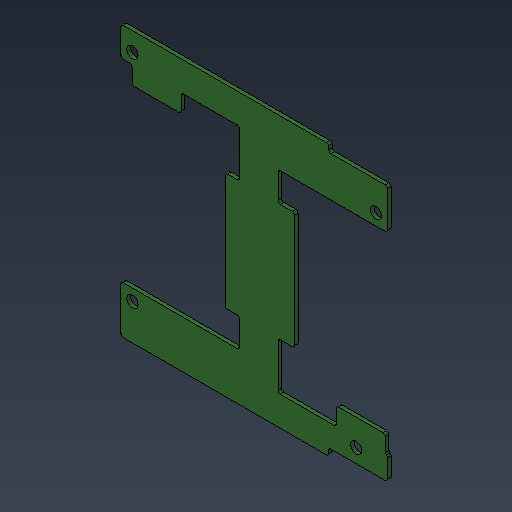
# Autodesk Inventor part: PCB_InterfaceBoard
Saved by Autodesk Inventor 2026.2 (Build 302298010, 298A)
## iProperties
Created: 2026-04-14
Part Number: PCB_InterfaceBoard
Material: Generic
Document SubType Name: Modeling
Designer: szymo
Density: 1 g/cm^3
Appearance: Default(1)
Mass: 1.18658 g
Surface Area: 32.671 cm^2
Volume: 1.18658 cm^3
Author: szymo
Autodesk Inventor part; units mm, degrees
ref_plane "YZ Plane" through (0, 0, 0) normal (1, 0, 0) x (0, 1, 0)
ref_plane "XZ Plane" through (0, 0, 0) normal (0, 1, 0) x (-1, 0, 0)
ref_plane "XY Plane" through (0, 0, 0) normal (0, 0, 1) x (1, 0, 0)
sketch "Sketch1" plane through (0, 0, 0) normal (0, 0, 1) x (1, 0, 0)
  line L0 (13.7023, 4) -> (22.3525, 4)
  line L1 (22.3525, 0) -> (59.3371, 0)
  line L2 (59.3371, 0) -> (59.3371, 9.3)
  line L3 (59.3371, 9.3) -> (0, 9.3)
  line L4 (0, 4) -> (0, 9.3)
  line L5 (0, 4) -> (2.4551, 4)
  line L6 (2.4551, 4) -> (2.4551, 0)
  line L7 (2.4551, 0) -> (13.7023, 0)
  line L8 (0, -38.4) -> (39.318, -38.4)
  line L9 (0, -38.4) -> (0, -47.7)
  line L10 (0, -47.7) -> (59.3371, -47.7)
  line L11 (59.3371, -42.4) -> (59.3371, -47.7)
  line L12 (59.3371, -42.4) -> (58.882, -42.4)
  line L13 (58.882, -42.4) -> (58.882, -38.4)
  line L14 (47.6348, -38.4) -> (58.882, -38.4)
  line L15 (47.6348, -42.4) -> (39.318, -42.4)
  line L16 (39.0735, -33.15) -> (39.0735, -5.25)
  line L17 (39.0735, -5.25) -> (39.9371, -5.25)
  line L18 (39.9371, -5.25) -> (39.9371, -33.15)
  line L19 (39.9371, -33.15) -> (39.0735, -33.15)
  line L20 (22.2636, -5.25) -> (22.2636, -33.15)
  line L21 (22.2636, -33.15) -> (21.4, -33.15)
  line L22 (21.4, -33.15) -> (21.4, -5.25)
  line L23 (21.4, -5.25) -> (22.2636, -5.25)
  line L24 (21.4, 0) -> (21.4, -38.4)
  line L25 (16.4787, 3) -> (18.0543, 3)
  line L26 (39.9371, -38.4) -> (39.9371, 0)
  line L27 (39.9371, 0) -> (62.3371, 0)
  line L28 (59.1371, 9.1) -> (59.1371, 0.2)
  line L29 (59.1371, 0.2) -> (34.9371, 0.2)
  line L30 (34.9371, 0.2) -> (34.9371, -6.25)
  line L31 (34.9371, -6.25) -> (38.5735, -6.25)
  line L32 (38.5735, -6.25) -> (38.5735, -32.15)
  line L33 (34.9371, -32.15) -> (34.9371, -42.6)
  line L34 (59.1371, -42.6) -> (59.1371, -47.5)
  line L35 (59.1371, -47.5) -> (46.1371, -47.5)
  line L36 (0.2, -49.1) -> (0.2, -38.6)
  line L37 (0.2, -38.6) -> (26.4, -38.6)
  line L38 (26.4, -38.6) -> (26.4, -32.15)
  line L39 (26.4, -32.15) -> (23.2636, -32.15)
  line L40 (23.2636, -32.15) -> (23.2636, -6.25)
  line L41 (23.2636, -6.25) -> (26.4, -6.25)
  line L42 (26.4, -6.25) -> (26.4, 4.2)
  line L43 (0.2, 4.2) -> (0.2, 9.1)
  line L44 (38.5735, -32.15) -> (34.9371, -32.15)
  circle A0 centre (2.75, -41.15) radius 1.75
  circle A1 centre (52.2136, -44.4) radius 1.75
  circle A2 centre (56.5871, 2.75) radius 1.75
  circle A3 centre (2.75, 6.55) radius 1.75
  circle A4 centre (56.5871, 2.75) radius 1.25
  circle A5 centre (52.2136, -44.4) radius 1.25
  circle A6 centre (2.75, -41.15) radius 1.25
  circle A7 centre (2.75, 6.55) radius 1.25
  line L45 (26.4, 4.2) -> (13.5023, 4.2)
  line L46 (13.5023, 4.2) -> (13.5023, 0.2)
  line L47 (13.5023, 0.2) -> (2.6551, 0.2)
  line L48 (2.6551, 0.2) -> (2.6551, 4.2)
  line L49 (2.6551, 4.2) -> (0.2, 4.2)
  line L50 (59.1371, -42.6) -> (58.682, -42.6)
  line L51 (58.682, -42.6) -> (58.682, -38.6)
  line L52 (58.682, -38.6) -> (47.8348, -38.6)
  line L53 (47.8348, -38.6) -> (47.8348, -42.6)
  line L54 (47.8348, -42.6) -> (34.9371, -42.6)
  line L55 (39.318, -42.4) -> (39.318, -38.4)
  line L56 (47.6348, -38.4) -> (47.6348, -42.4)
  line L57 (13.7023, 0) -> (13.7023, 4)
  line L58 (22.3525, 4) -> (22.3525, 0)
  spline S0 degree 2 poles (41.0471, 11.3) (40.5342, 11.2191) (40.0213, 11.3) knots 0 0 0 1 1 1 weights 1 1.01269 1
  line L59 (0, 11.3) -> (40.0213, 11.3)
  line L60 (0, 9.3) -> (0, 11.3)
  line L61 (0, 9.3) -> (46.3371, 9.3)
  line L62 (46.3371, 9.3) -> (46.3371, 11.3)
  line L63 (41.0471, 11.3) -> (46.3371, 11.3)
  spline S1 degree 2 poles (20.1962, -49.7) (20.5821, -49.6542) (20.9681, -49.7) knots 0 0 0 1 1 1 weights 1 1.007125 1
  line L64 (46.3371, -49.7) -> (20.9681, -49.7)
  line L65 (46.3371, -47.7) -> (46.3371, -49.7)
  line L66 (0, -47.7) -> (46.3371, -47.7)
  line L67 (0, -47.7) -> (0, -49.7)
  line L68 (20.1962, -49.7) -> (0, -49.7)
  line L69 (46.1371, -49.1) -> (0.2, -49.1)
  line L70 (46.1371, -47.5) -> (46.1371, -49.1)
  line L71 (46.1371, 9.1) -> (59.1371, 9.1)
  line L72 (46.1371, 9.1) -> (46.1371, 10.7)
  line L73 (46.1371, 10.7) -> (0.2, 10.7)
  line L74 (0.2, 10.7) -> (0.2, 9.1)
  point P0 (0, 0)
  point P1 (34.9371, 0)
  point P2 (34.9371, -38.4)
  dimension "d1" = 0.2
  dimension "d3" = 0.2
  dimension "d5" = 0.2
  dimension "d7" = 0.2
  dimension "d8" = 0.2
  dimension "d10" = 0.2
  dimension "d11" = 0.2
  dimension "d16" = 1
  dimension "d17" = 0.5
  dimension "d18" = 5
  dimension "d19" = 1
  dimension "d20" = 1
  dimension "d21" = 1
  dimension "d22" = 1
  dimension "d23" = 5
  dimension "d24" = 5
  dimension "d25" = 5
  dimension "d29" = 2.5
  dimension "d30" = 2.5
  dimension "d31" = 2.5
  dimension "d32" = 2.5
  dimension "d33" = 0.2
  dimension "d34" = 0.2
  dimension "d35" = 0.2
  dimension "d37" = 0.2
  dimension "d38" = 0.2
  dimension "d40" = 0.2
  dimension "d41" = 0.2
  dimension "d42" = 0.2
  dimension "d43" = 0.2
  dimension "d44" = 0.2
  dimension "d45" = 0.6
  dimension "d46" = 0.2
  dimension "d47" = 0.2
  dimension "d48" = 0.2
  dimension "d49" = 0.6
  constraints: 91 end point, 19 perpendicular, 11 vertical, 9 horizontal, 4 centre point, 4 coincident, 3 parallel, 14 other
  measures "d1" distance between parallel lines of L29 L27
  measures "d3" distance between parallel lines of L2 L28
  measures "d5" distance between parallel lines of L4 L43
  measures "d7" distance between parallel lines of L8 L37
  measures "d8" distance between parallel lines of L9 L36
  measures "d10" distance between parallel lines of L11 L34
  measures "d11" distance between parallel lines of L10 L35
  measures "d16" distance between parallel lines of L40 L20
  measures "d17" distance between parallel lines of L16 L32
  measures "d18" distance between parallel lines of L42 L24
  measures "d19" distance between parallel lines of L41 L23
  measures "d20" distance between parallel lines of L31 L17
  measures "d21" distance between parallel lines of L39 L21
  measures "d22" distance between parallel lines of L19 L44
  measures "d23" distance between parallel lines of L30 L26
  measures "d24" distance between parallel lines of L33 L26
  measures "d25" distance between parallel lines of L24 L38
  measures "d29" diameter of A4
  measures "d30" diameter of A5
  measures "d31" diameter of A6
  measures "d32" diameter of A7
  measures "d33" distance between parallel lines of L5 L49
  measures "d34" distance between parallel lines of L48 L6
  measures "d35" distance between parallel lines of L7 L47
  measures "d37" distance between parallel lines of L45 L0
  measures "d38" distance between parallel lines of L54 L15
  measures "d40" distance between parallel lines of L14 L52
  measures "d41" distance between parallel lines of L51 L13
  measures "d42" distance between parallel lines of L12 L50
  measures "d43" distance between parallel lines of L53 L56
  measures "d44" distance between parallel lines of L65 L70
  measures "d45" distance between parallel lines of L68 L69
  measures "d46" distance between parallel lines of L57 L46
  measures "d47" distance between parallel lines of L3 L71
  measures "d48" distance between parallel lines of L62 L72
  measures "d49" distance between parallel lines of L59 L73
extrude "Extrusion1" add sketch "Sketch1" along normal blind 0.8 contours L42 L45 L46 L47 L48 L49 L43 L74 L3 L72 L71 L28 L29 L30 L1 | L1 L30 L31 L32 L44 L33 L8 L38 L39 L40 L41 L42 | L74 L73 L72 L3 | L8 L33 L54 L53 L52 L51 L50 L34 L35 L70 L10 L36 L37 L38 | L10 L70 L69 L36 | A0 | A1 | A2 | A3
fillet "Fillet1" radius 0.5 32 edges at (59.1371, -47.5, 0.4) (59.1371, -42.6, 0.4) (0.2, -38.6, 0.4) (26.4, -38.6, 0.4) (26.4, -32.15, 0.4) (23.2636, -32.15, 0.4) (23.2636, -6.25, 0.4) (26.4, -6.25, 0.4) (26.4, 4.2, 0.4) (0.2, 4.2, 0.4) (59.1371, 9.1, 0.4) (59.1371, 0.2, 0.4) (34.9371, 0.2, 0.4) (34.9371, -6.25, 0.4) (38.5735, -6.25, 0.4) (38.5735, -32.15, 0.4) (34.9371, -32.15, 0.4) (34.9371, -42.6, 0.4) (2.6551, 4.2, 0.4) (2.6551, 0.2, 0.4) (13.5023, 4.2, 0.4) (13.5023, 0.2, 0.4) (47.8348, -42.6, 0.4) (47.8348, -38.6, 0.4) (58.682, -38.6, 0.4) (58.682, -42.6, 0.4) (46.1371, -47.5, 0.4) (46.1371, -49.1, 0.4) (0.2, -49.1, 0.4) (46.1371, 9.1, 0.4) (46.1371, 10.7, 0.4) (0.2, 10.7, 0.4)
equation "\"d5\" = d1"
equation "\"d7\" = d1"
equation "\"d8\" = d1"
equation "\"d10\" = d1"
equation "\"d11\" = d1"
equation "\"d18\" = d23"
equation "\"d19\" = d20"
equation "\"d21\" = d20"
equation "\"d22\" = d20"
equation "\"d24\" = d23"
equation "\"d25\" = d23"
equation "\"d30\" = d29"
equation "\"d31\" = d29"
equation "\"d32\" = d29"
equation "\"d33\" = d1"
equation "\"d34\" = d1"
equation "\"d35\" = d1"
equation "\"d37\" = d1"
equation "\"d38\" = d1"
equation "\"d40\" = d1"
equation "\"d41\" = d1"
body "Solid1"
